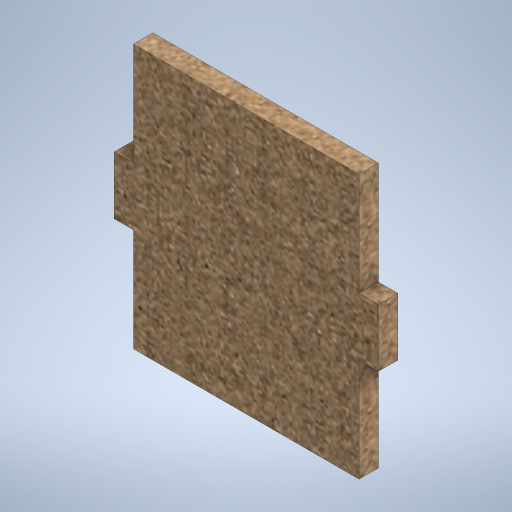
# Autodesk Inventor part: Wall_Base1
Saved by Autodesk Inventor 2024 (Build 280153000, 153)
## iProperties
Created: 2023-11-23
Part Number: Wall_Base1
Material: MDF Tablero de fibras de densidad media
Document SubType Name: Modeling
Designer: marco
Density: 0.8 g/cm^3
Appearance: Cartón - Ondulado
Author: marco
Autodesk Inventor part; units mm, degrees
ref_plane "YZ Plane" through (0, 0, 0) normal (1, 0, 0) x (0, 1, 0)
ref_plane "XZ Plane" through (0, 0, 0) normal (0, 1, 0) x (-1, 0, 0)
ref_plane "XY Plane" through (0, 0, 0) normal (0, 0, 1) x (1, 0, 0)
sketch "Boceto1" plane through (0, 0, 0) normal (0, 0, 1) x (1, 0, 0)
  line L0 (17.5, 22) -> (17.5, 6)
  line L1 (17.5, 6) -> (20.5, 6)
  line L2 (20.5, 6) -> (20.5, -3)
  line L3 (20.5, -3) -> (17.5, -3)
  line L4 (17.5, -3) -> (17.5, -19)
  line L5 (17.5, -19) -> (-17.5, -19)
  line L6 (-17.5, -19) -> (-17.5, -3)
  line L7 (-17.5, -3) -> (-20.5, -3)
  line L8 (-20.5, 0) -> (-20.5, -3)
  line L9 (-20.5, 6) -> (-20.5, -3)
  line L10 (-17.5, 6) -> (-17.5, 22)
  line L11 (-17.5, 22) -> (17.5, 22)
  line L12 (-20.5, 6) -> (-17.5, 6)
  constraints: 26 end point
extrude "Extrusión1" add sketch "Boceto1" along normal blind 3
